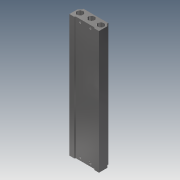
# Autodesk Inventor part: manifold-block
Saved by Autodesk Inventor 2017 (Build 210142000, 142)
## iProperties
Created: 2018-06-21
Part Number: manifold-block
Material: Steel, Alloy
Document SubType Name: Modeling
Designer: Luiz Gustavo
Density: 7.73 g/cm^3
Appearance: Semi-Polished
Author: Luiz Gustavo
Autodesk Inventor part; units mm, degrees
ref_plane "YZ Plane" through (0, 0, 0) normal (1, 0, 0) x (0, 1, 0)
ref_plane "XZ Plane" through (0, 0, 0) normal (0, 1, 0) x (-1, 0, 0)
ref_plane "XY Plane" through (0, 0, 0) normal (0, 0, 1) x (1, 0, 0)
sketch "Sketch1" plane through (0, 0, 0) normal (0, 0, 1) x (1, 0, 0)
  circle A0 centre (0, 0) radius 6.35
  line L0 (0, 9) -> (-25.5, 9)
  line L1 (-25.5, 9) -> (-25.5, 7)
  line L2 (-25.5, 7) -> (-30, 2.5)
  line L3 (-30, 2.5) -> (-30, -15)
  line L4 (-30, -15) -> (-21, -15)
  line L5 (-21, -15) -> (-19, -13)
  line L6 (-19, -13) -> (0, -13)
  line L7 (0, 9) -> (0, -13) construction
  line L8 (0, 9) -> (25.5, 9)
  line L9 (25.5, 9) -> (25.5, 7)
  line L10 (25.5, 7) -> (30, 2.5)
  line L11 (30, 2.5) -> (30, -15)
  line L12 (30, -15) -> (21, -15)
  line L13 (21, -15) -> (19, -13)
  line L14 (19, -13) -> (0, -13)
  circle A1 centre (-21.5, -2) radius 6.35
  circle A2 centre (21.5, -2) radius 6.35
  dimension "d0" = 12.7
  dimension "d1" = 43
  dimension "d2" = 60
  dimension "d3" = 51
  dimension "d4" = 13
  dimension "d5" = 24
  dimension "d6" = 38
  dimension "d7" = 2
  dimension "d8" = 135
  dimension "d9" = 2
  dimension "d10" = 2
  constraints: 30 end point, 6 symmetric about line, 3 centre point, 3 parallel, 2 perpendicular, 1 coincident, 1 equal radius, 1 horizontal, 1 point on line, 1 vertical, 1 other
  measures "d0" diameter of A0
  measures "d1" distance of A1.centre A2.centre
  measures "d2" distance between parallel lines of L11 L3
  measures "d3" distance between parallel lines of L9 L1
  measures "d4" distance from line of L12 A2.centre
  measures "d5" distance between parallel lines of L12 L8
  measures "d6" distance of L5.end L13.end
  measures "d7" distance of L8.end L9.end
  measures "d8" angle of L3 L2
  measures "d9" vertical distance of A0.centre A1.centre
  measures "d10" distance between parallel lines of L12 L14
extrude "Extrusion1" add sketch "Sketch1" along normal mid plane 253
sketch "Sketch2" plane through (-25.5, 9, 126.5) normal (0, 1, 0) x (1, 0, 0)
  line L0 (0, 253) -> (0, 0) projected
  line L1 (51, 0) -> (0, 0) projected
  line L2 (51, 253) -> (51, 0) projected
  line L3 (0, 253) -> (51, 253) projected
  line L4 (51, 0) -> (0, 0) construction
  line L5 (25.5, 0) -> (25.5, 253) construction
  line L6 (0, 126.5) -> (51, 126.5) construction
  circle A0 centre (15, 6) radius 2.25
  circle A1 centre (36, 6) radius 2.25
  circle A2 centre (25.5, 23) radius 6.35
  circle A3 centre (7.5, 23) radius 3.175
  circle A4 centre (43.5, 23) radius 3.175
  line L7 (43.5, 23) -> (7.5, 23) construction
  circle A5 centre (6.5, 31.5) radius 1.6
  circle A6 centre (44.5, 14.5) radius 1.6
  circle A7 centre (6.5, 54.5) radius 1.6
  circle A8 centre (7.5, 46) radius 3.175
  circle A9 centre (25.5, 46) radius 6.35
  circle A10 centre (43.5, 46) radius 3.175
  circle A11 centre (44.5, 37.5) radius 1.6
  circle A12 centre (6.5, 77.5) radius 1.6
  circle A13 centre (7.5, 69) radius 3.175
  circle A14 centre (25.5, 69) radius 6.35
  circle A15 centre (43.5, 69) radius 3.175
  circle A16 centre (44.5, 60.5) radius 1.6
  circle A17 centre (6.5, 100.5) radius 1.6
  circle A18 centre (7.5, 92) radius 3.175
  circle A19 centre (25.5, 92) radius 6.35
  circle A20 centre (43.5, 92) radius 3.175
  circle A21 centre (44.5, 83.5) radius 1.6
  circle A22 centre (6.5, 123.5) radius 1.6
  circle A23 centre (7.5, 115) radius 3.175
  circle A24 centre (25.5, 115) radius 6.35
  circle A25 centre (43.5, 115) radius 3.175
  circle A26 centre (44.5, 106.5) radius 1.6
  circle A27 centre (6.5, 146.5) radius 1.6
  circle A28 centre (7.5, 138) radius 3.175
  circle A29 centre (25.5, 138) radius 6.35
  circle A30 centre (43.5, 138) radius 3.175
  circle A31 centre (44.5, 129.5) radius 1.6
  circle A32 centre (6.5, 169.5) radius 1.6
  circle A33 centre (7.5, 161) radius 3.175
  circle A34 centre (25.5, 161) radius 6.35
  circle A35 centre (43.5, 161) radius 3.175
  circle A36 centre (44.5, 152.5) radius 1.6
  circle A37 centre (6.5, 192.5) radius 1.6
  circle A38 centre (7.5, 184) radius 3.175
  circle A39 centre (25.5, 184) radius 6.35
  circle A40 centre (43.5, 184) radius 3.175
  circle A41 centre (44.5, 175.5) radius 1.6
  circle A42 centre (6.5, 215.5) radius 1.6
  circle A43 centre (7.5, 207) radius 3.175
  circle A44 centre (25.5, 207) radius 6.35
  circle A45 centre (43.5, 207) radius 3.175
  circle A46 centre (44.5, 198.5) radius 1.6
  circle A47 centre (6.5, 238.5) radius 1.6
  circle A48 centre (7.5, 230) radius 3.175
  circle A49 centre (25.5, 230) radius 6.35
  circle A50 centre (43.5, 230) radius 3.175
  circle A51 centre (44.5, 221.5) radius 1.6
  circle A52 centre (15, 247) radius 2.25
  circle A53 centre (36, 247) radius 2.25
  point P0 (25.5, 126.5)
  dimension "d13" = 4.5
  dimension "d14" = 21
  dimension "d15" = 6
  dimension "d16" = 12.7
  dimension "d17" = 6.35
  dimension "d18" = 36
  dimension "d19" = 23
  dimension "d21" = 38
  dimension "d22" = 3.2
  dimension "d23" = 19
  dimension "d27" = 23
  dimension "d38" = 17
  dimension "d39" = 8.5
  constraints: 54 centre point, 6 end point, 5 midpoint, 2 equal radius, 2 symmetric about line, 1 horizontal, 1 perpendicular, 1 point on line, 1 vertical, 94 other
  measures "d13" diameter of A0
  measures "d14" distance of A1.centre A0.centre
  measures "d15" distance from line of L1 A0.centre
  measures "d16" diameter of A2
  measures "d17" diameter of A4
  measures "d18" distance of L7.end L7.start
  measures "d19" distance between parallel lines of L1 L7
  measures "d21" horizontal distance of A6.centre A5.centre
  measures "d22" diameter of A5
  measures "d23" distance from line of L5 A5.centre
  measures "d27" distance of A5.centre A7.centre
  measures "d38" vertical distance of A6.centre A5.centre
  measures "d39" distance from line of L7 A5.centre
extrude "Extrusion2" cut sketch "Sketch2" against normal through all contours A0 | A1 | A52 | A53
extrude "Extrusion3" cut sketch "Sketch2" against normal blind 15 contours A2 | A3 | A4 | A8 | A9 | A10 | A13 | A14 | A15 | A18 | A19 | A20 | A23 | A24 | A25 | A28 | A29 | A30 | A33 | A34 | A35 | A38 | A39 | A40 | A43 | A44 | A45 | A48 | A49 | A50
extrude "Extrusion4" cut sketch "Sketch2" against normal blind 5 contours A5 | A6 | A7 | A11 | A12 | A16 | A17 | A21 | A22 | A26 | A27 | A31 | A32 | A36 | A37 | A41 | A42 | A46 | A47 | A51
equation "\"d23\" = 0.5 * d21"
equation "\"d39\" = 0.5 * d38"
body "Solid1"
